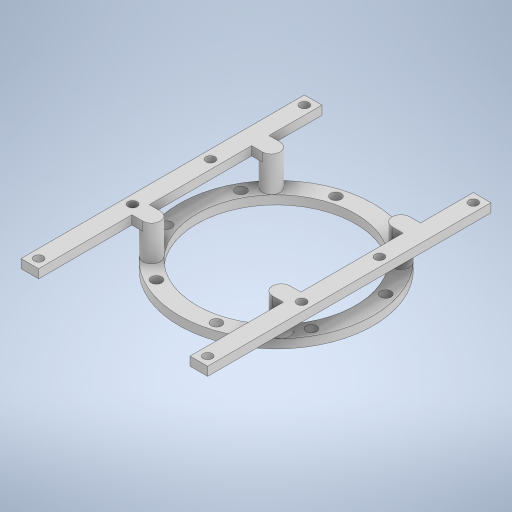
# Autodesk Inventor part: grumpy mount
Saved by Autodesk Inventor 2023 (Build 270158000, 158)
## iProperties
Created: 2022-09-06
Part Number: grumpy mount
Material: Generic
Document SubType Name: Modeling
Designer: Eli
Density: 1 g/cm^3
Appearance: Default
Author: Eli
Autodesk Inventor part; units mm, degrees
ref_plane "YZ Plane" through (0, 0, 0) normal (1, 0, 0) x (0, 1, 0)
ref_plane "XZ Plane" through (0, 0, 0) normal (0, 1, 0) x (-1, 0, 0)
ref_plane "XY Plane" through (0, 0, 0) normal (0, 0, 1) x (1, 0, 0)
sketch "Sketch1" plane through (0, 0, 0) normal (0, 1, 0) x (-1, 0, 0)
  circle A0 centre (0, 0) radius 31.8262 construction
  circle A1 centre (27.9401, -15.24) radius 1.905
  line L0 (31.8262, 0) -> (0, 0) construction
  circle A2 centre (0, 0) radius 31.8262 construction
  circle A3 centre (30.5329, 8.9803) radius 1.905
  circle A4 centre (0, 0) radius 31.8262 construction
  circle A5 centre (15.24, 27.9401) radius 1.905
  circle A6 centre (0, 0) radius 31.8262 construction
  circle A7 centre (-8.9803, 30.5329) radius 1.905
  circle A8 centre (0, 0) radius 31.8262 construction
  circle A9 centre (-27.9401, 15.24) radius 1.905
  circle A10 centre (0, 0) radius 31.8262 construction
  circle A11 centre (-30.5329, -8.9803) radius 1.905
  circle A12 centre (0, 0) radius 31.8262 construction
  circle A13 centre (-15.24, -27.9401) radius 1.905
  circle A14 centre (0, 0) radius 31.8262 construction
  circle A15 centre (8.9803, -30.5329) radius 1.905
  circle A16 centre (0, 0) radius 35.0012
  circle A17 centre (0, 0) radius 28.6512
  point P0 (22.5045, 22.5045)
  point P1 (0, 31.8262)
  point P2 (-22.5045, 22.5045)
  point P3 (-31.8262, 0)
  point P4 (-22.5045, -22.5045)
  point P5 (0, -31.8262)
  point P6 (22.5045, -22.5045)
  dimension "d0" = 63.6524
  dimension "d1" = 3.81
  dimension "d2" = 15.24
  dimension "d5" = 360
  dimension "d7" = 70.0024
  dimension "d8" = 57.3024
  constraints: 18 centre point, 16 point on circle, 3 coincident, 2 end point, 1 horizontal, 41 other
  measures "d0" diameter of A0
  measures "d1" diameter of A1
  measures "d2" distance from line of L0 A1.centre
  measures "d7" diameter of A16
  measures "d8" diameter of A17
extrude "Extrusion2" add sketch "Sketch1" along normal blind 3.175
sketch "Sketch3" plane through (0, 3.175, 0) normal (0, 1, 0) x (1, 0, 0)
  circle A0 centre (-30.5329, -8.9803) radius 1.905 construction
  line L0 (-32.4379, -8.9803) -> (-30.5329, -8.9803) construction
  line L1 (-28.6279, 0) -> (0, 0) construction
  line L2 (0, 0) -> (0, -28.6565) construction
  circle A1 centre (0, 0) radius 31.8262 construction
  circle A2 centre (-23.3832, -21.5901) radius 3.175
  circle A3 centre (0, 0) radius 28.6512 projected
  circle A4 centre (-23.3832, 21.5901) radius 3.175
  circle A5 centre (23.3832, -21.5901) radius 3.175
  circle A6 centre (23.3832, 21.5901) radius 3.175
  circle A7 centre (-15.24, -27.9401) radius 1.905 construction
  line L3 (-15.24, -27.9401) -> (-17.145, -27.9401) construction
  circle A8 centre (-27.9401, 15.24) radius 1.905 construction
  line L4 (-29.8451, 15.24) -> (-27.9401, 15.24) construction
  dimension "d14" = 6.35
  dimension "d15" = 6.3501
  constraints: 10 end point, 5 centre point, 4 horizontal, 3 horizontal alignment, 3 symmetric about line, 2 point on circle, 1 coincident, 1 perpendicular, 1 tangent, 6 other
  measures "d14" vertical distance of A2.centre L3.start
  measures "d15" vertical distance of A4.centre L4.end
extrude "Extrusion3" add sketch "Sketch3" along normal blind 9.525 contours A2 | A4 | A6 | A5
sketch "Sketch7" plane through (-23.3832, 12.7, -21.5901) normal (0, 1, 0) x (1, 0, 0)
  circle A0 centre (-7.0968, 19.0499) radius 1.651
  circle A1 centre (53.8632, 19.0499) radius 1.651
  line L0 (-7.0968, 19.0499) -> (53.8632, 19.0499) construction
  circle A2 centre (0, 0) radius 3.175 construction
  arc A3 (49.0991, 2.1538) -> (44.4337, -2.1538) centre (46.7664, 0) ccw construction
  line L1 (0, 0) -> (46.7664, 0) construction
  line L2 (23.3832, 0) -> (23.3832, -21.5901) construction
  circle A4 centre (-7.0968, -14.8464) radius 1.651
  circle A5 centre (53.8632, -14.8464) radius 1.651
  line L3 (-7.0968, -14.8464) -> (53.8632, -14.8464) construction
  circle A6 centre (-7.0968, -42.9134) radius 1.651
  circle A7 centre (53.8632, -42.9134) radius 1.651
  line L4 (-7.0968, -42.9134) -> (53.8632, -42.9134) construction
  circle A8 centre (-7.0968, -76.8097) radius 1.651
  circle A9 centre (53.8632, -76.8097) radius 1.651
  line L5 (-7.0968, -76.8097) -> (53.8632, -76.8097) construction
  circle A10 centre (-4.5569, -6.3501) radius 1.905 construction
  line L6 (-4.5569, -6.3501) -> (23.3832, -6.3501) construction
  line L7 (-10.2718, 22.2249) -> (-3.9218, 22.2249)
  line L8 (-3.9218, 22.2249) -> (-3.9218, -79.9847)
  line L9 (-3.9218, -79.9847) -> (-10.2718, -79.9847)
  line L10 (-10.2718, -79.9847) -> (-10.2718, 22.2249)
  line L11 (-7.0968, 20.7009) -> (-7.0968, 19.0499) construction
  line L12 (-3.9218, 3.175) -> (0, 3.175)
  line L13 (3.175, 0) -> (3.175, 0)
  line L14 (0, -3.175) -> (-3.9218, -3.175)
  line L15 (-3.9218, -3.175) -> (-3.9218, 3.175)
  line L16 (-3.9218, -40.0052) -> (0, -40.0052)
  line L17 (3.175, -43.1802) -> (3.175, -43.1802)
  line L18 (0, -46.3552) -> (-3.9218, -46.3552)
  line L19 (-3.9218, -46.3552) -> (-3.9218, -40.0052)
  circle A11 centre (0, -43.1802) radius 3.175 projected
  arc A12 (3.175, 0) -> (0, 3.175) centre (0, 0) ccw
  arc A13 (0, -3.175) -> (3.175, 0) centre (0, 0) ccw
  arc A14 (3.175, -43.1802) -> (0, -40.0052) centre (0, -43.1802) ccw
  arc A15 (0, -46.3552) -> (3.175, -43.1802) centre (0, -43.1802) ccw
  circle A16 centre (46.7664, 0) radius 3.175 construction
  line L20 (57.0382, 22.2249) -> (50.6882, 22.2249)
  line L21 (50.6882, 22.2249) -> (50.6882, -79.9847)
  line L22 (50.6882, -79.9847) -> (57.0382, -79.9847)
  line L23 (57.0382, -79.9847) -> (57.0382, 22.2249)
  line L24 (50.6882, 3.175) -> (46.7664, 3.175)
  line L25 (46.7664, -3.175) -> (50.6882, -3.175)
  line L26 (50.6882, -40.0052) -> (46.7664, -40.0052)
  line L27 (46.7664, -46.3552) -> (50.6882, -46.3552)
  circle A17 centre (46.7664, -43.1802) radius 3.175
  arc A18 (46.7664, 3.175) -> (43.5914, 0) centre (46.7664, 0) ccw
  arc A19 (43.5914, 0) -> (46.7664, -3.175) centre (46.7664, 0) ccw
  arc A20 (46.7664, -40.0052) -> (43.5914, -43.1802) centre (46.7664, -43.1802) ccw
  point P0 (-3.9218, -46.3552)
  point P1 (0, -46.3552)
  point P2 (0, -40.0052)
  point P3 (-3.9218, -3.175)
  point P4 (3.175, 0)
  point P5 (43.5914, 0)
  dimension "d22" = 3.302
  dimension "d23" = 60.96
  dimension "d24" = 3.302
  dimension "d25" = 60.96
  dimension "d26" = 33.8963
  dimension "d27" = 3.302
  dimension "d28" = 60.96
  dimension "d29" = 3.302
  dimension "d30" = 60.96
  dimension "d31" = 33.8963
  dimension "d32" = 28.067
  dimension "d33" = 25.4
  dimension "d34" = 6.35
  dimension "d35" = 3.175
  dimension "d36" = 3.175
  dimension "d37" = 3.175
  constraints: 56 end point, 23 symmetric about line, 16 centre point, 14 point on circle, 14 tangent, 7 horizontal, 6 parallel, 5 point on line, 4 coincident, 4 perpendicular, 2 equal radius, 2 vertical, 1 concentric, 1 midpoint, 1 vertical alignment, 12 other
  measures "d23" distance of A1.centre L0.start
  measures "d24" diameter of A4
  measures "d25" distance of A5.centre L3.start
  measures "d26" distance between parallel lines of L3 L0
  measures "d27" diameter of A6
  measures "d28" distance of A7.centre L4.start
  measures "d29" diameter of A8
  measures "d30" distance of A9.centre L5.start
  measures "d31" distance between parallel lines of L5 L4
  measures "d32" distance between parallel lines of L4 L3
  measures "d33" distance between parallel lines of L6 L0
  measures "d34" distance of L7.start L7.end
  measures "d35" distance from line of L7 L0.start
  measures "d36" distance from line of L9 L5.start
  measures "d37" radius of A12
extrude "Extrusion4" add sketch "Sketch7" along normal blind 3.175
body "Solid2"
